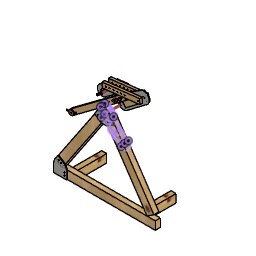
trebuchetAbril2025-Comps-v14 (Autodesk Fusion 360 design; units mm, degrees)
Autodesk Fusion 360 part; units mm, degrees
sketch "Boceto1" plane through (0, 0, 0) normal (0, 1, 0) x (1, 0, 0)
  line L0 (0, 0) -> (800, 0)
  line L1 (800, 0) -> (800, -65)
  line L2 (800, -65) -> (0, -65)
  line L3 (0, -65) -> (0, 0)
  line L4 (65, -65) -> (11.0416, -101.2421)
  line L5 (11.0416, -101.2421) -> (346.0416, -600)
  line L6 (346.0416, -600) -> (400, -563.7579)
  line L7 (400, -563.7579) -> (65, -65)
  line L8 (400, -65) -> (400, -814.7685) construction
  line L9 (400, -563.7579) -> (735, -65)
  line L10 (735, -65) -> (788.9584, -101.2421)
  line L11 (788.9584, -101.2421) -> (453.9584, -600)
  line L12 (453.9584, -600) -> (400, -563.7579)
  dimension "grosor3p" = 65
  dimension "d4" = 65
  dimension "d5" = 600
  dimension "d6" = 65
  dimension "tolerancia" = 1
  dimension "eje" = 10
  dimension "grosorR1b" = 20
  dimension "separacionAgujeros" = 30
  dimension "agujeroAjuste" = 10
  dimension "grosorR2" = 30
  dimension "agujeroTornillos" = 4
  constraint horizontal L0
  constraint vertical L1
  constraint horizontal L2
  constraint vertical L3
  constraint coincident L0.start L3.end
  constraint perpendicular L4 L5
  constraint parallel L4 L6
  constraint parallel L5 L7
  constraint coincident L2 L4.start
  constraint midpoint L2 L8.start
  constraint perpendicular L2 L8
  constraint coincident L6.end L8
  constraint symmetric L4.start L8 L9.end
  constraint symmetric L4.end L8 L10.end
  constraint symmetric L5.end L8 L11.end
  constraint symmetric L6.end L8 L7.start
  measures "grosor3p" distance of L0.start L2.end
  measures "d4" distance of L5 L7
  measures "d5" distance of L0 L5.end
  measures "d6" distance of L2.end L4.start
sketch "Boceto2" plane through (0, 0, 0) normal (0, 1, 0) x (1, 0, 0)
  line L0 (-333.2779, 0) -> (-245.9669, 0)
  line L1 (-245.9669, 0) -> (-245.9669, -600)
  line L2 (-245.9669, -600) -> (-333.2779, -600)
  line L3 (-333.2779, -600) -> (-333.2779, 0)
  constraint horizontal L0
  constraint vertical L1
  constraint horizontal L2
  constraint vertical L3
extrude "Extruir1" add sketch "Boceto1" along normal blind 40 contours L0 L1 L2 L3 | L4 L5 L6 L7 | L9 L10 L11 L12 makes body 1
sketch "Boceto3" plane through (0, 0, 0) normal (0, -1, 0) x (1, 0, 0)
  line L0 (65, 65) -> (400, 563.7579)
  line L1 (400, 563.7579) -> (346.0416, 600)
  line L2 (346.0416, 600) -> (11.0416, 101.2421)
  line L3 (11.0416, 101.2421) -> (65, 65)
  circle A0 centre (65, 65) radius 65
  line L4 (0, 0) -> (105, 0)
  line L5 (105, 0) -> (105, 63.8522)
  line L6 (105, 63.8522) -> (0, 63.8522)
  line L7 (0, 63.8522) -> (0, 0)
  line L8 (65, 65) -> (11.0416, 101.2421)
  line L9 (11.0416, 101.2421) -> (33.3445, 134.4473)
  line L10 (33.3445, 134.4473) -> (87.3029, 98.2052)
  line L11 (87.3029, 98.2052) -> (65, 65)
  circle A1 centre (400, 600) radius 44.7924
  line L12 (0, 0) -> (800, 0)
  line L13 (788.9584, 101.2421) -> (453.9584, 600)
  line L14 (323.7388, 566.7948) -> (377.6971, 530.5527)
  line L15 (377.6971, 530.5527) -> (416.7749, 588.7328)
  line L16 (416.7749, 588.7328) -> (362.8165, 624.975)
  line L17 (362.8165, 624.975) -> (323.7388, 566.7948)
  line L18 (422.7884, 530.8788) -> (476.2612, 566.7948)
  line L19 (476.2612, 566.7948) -> (437.1835, 624.975)
  line L20 (437.1835, 624.975) -> (383.7107, 589.059)
  line L21 (383.7107, 589.059) -> (422.7884, 530.8788)
  line L22 (87.3029, 98.2052) -> (105, 63.8522)
  line L23 (377.6971, 530.5527) -> (422.7884, 530.8788)
  dimension "traslape" = 40
  dimension "d10" = 40
  dimension "d11" = 600
  dimension "d12" = 40
  dimension "d13" = 40
  constraint coincident L0.start L3.end
  constraint coincident L2.end A0
  constraint horizontal L4
  constraint vertical L5
  constraint horizontal L6
  constraint vertical L7
  constraint coincident L4.start L7.end
  constraint perpendicular L8 L9
  constraint parallel L8 L10
  constraint parallel L9 L11
  constraint coincident L2.end L3.start
  constraint perpendicular L2 L8
  constraint vertical L0.end A1.centre
  constraint tangent A1 L13
  constraint perpendicular L14 L15
  constraint parallel L14 L16
  constraint parallel L15 L17
  constraint coincident L0 L14.end
  constraint perpendicular L0 L14
  constraint coincident L2 L14.start
  constraint perpendicular L18 L19
  constraint parallel L18 L20
  constraint parallel L19 L21
  constraint coincident L13 L18.end
  constraint perpendicular L13 L18
  constraint coincident A1 L16.end
  constraint coincident A1 L19.end
  measures "traslape" distance of L8 L10
  measures "d10" distance of L0.start L5
  measures "d11" distance of A1.centre L12
  measures "d12" distance of L13.end L18
  measures "d13" distance of L1 L14
extrude "Extruir2" add sketch "Boceto3" along normal blind 6 separate body contours L0 L3 A0 L8 L10 L11 | L0 L3 A0 L6 L8 L11 L22 | L2 A0 L9 L10 | A0 L5 L6 | A0 L4 L6 L7 L12 | L0 L1 L2 A1 L14 L15 L17 | L0 A1 L15 L21 L23 | A0 L4 L5 L12 | L0 L1 A1 L15 | L0 A1 L15 L21 | A1 L13 L18 L19 L21 | L1 A1 L17 | L1 A1 L15 L16 L20 L21 | A1 L15 L16 L20 L21 | A1 L16 L20 | L15 L16 L20 L21 makes body 2 at (35.0034, 0, 21.2841) makes body 3 at (407.5961, 0, 593.6096)
sketch "Boceto4" plane through (0, 40, 0) normal (0, 1, 0) x (-1, 0, 0)
  line L0 (0, 65) -> (-65, 65)
  line L1 (-65, 65) -> (-735, 65)
  line L2 (-735, 65) -> (-800, 65)
  line L3 (-800, 65) -> (-800, 0)
  line L4 (-800, 0) -> (0, 0)
  line L5 (0, 0) -> (0, 65)
  line L6 (-145, 0) -> (-105, 0)
  line L7 (-105, 0) -> (-105, 65)
  line L8 (-105, 65) -> (-145, 65)
  line L9 (-145, 65) -> (-145, 0)
  line L10 (-400, 65) -> (-400, 691.7695) construction
  line L11 (-655, 65) -> (-655, 0)
  line L12 (-695, 65) -> (-655, 65)
  line L13 (-695, 0) -> (-695, 65)
  line L14 (-655, 0) -> (-695, 0)
  dimension "d16" = 40
  dimension "d17" = 105
  constraint horizontal L6
  constraint vertical L7
  constraint horizontal L8
  constraint vertical L9
  constraint coincident L1 L7.end
  constraint coincident L4 L6.start
  constraint midpoint L1 L10.start
  constraint perpendicular L1 L10
  constraint symmetric L6.start L10 L11.end
  constraint symmetric L6.end L10 L13.start
  constraint symmetric L7.end L10 L12.start
  constraint symmetric L8.end L10 L11.start
  measures "d16" distance of L7.end L8.end
  measures "d17" distance of L5 L7
sketch "Boceto5" plane through (0, 0, 0) normal (0, 0, 1) x (1, 0, 0)
  line L0 (-250, 0) -> (-340.1586, 0)
  line L1 (-340.1586, 0) -> (-340.1586, 310)
  line L2 (-340.1586, 310) -> (-250, 310)
  line L3 (-250, 310) -> (-250, 0)
  dimension "base" = 310
  constraint horizontal L0
  constraint vertical L1
  constraint horizontal L2
  constraint vertical L3
  measures "base" distance of L0.end L1.end
extrude "Extruir3" add sketch "Boceto4" along normal blind 230 separate body contours L1 L4 L6 L7 L8 L9 | L1 L4 L11 L12 L13 L14 makes body 4 at (105, 116.6667, 21.6667) makes body 5 at (655, 116.6667, 43.3333)
sketch "Boceto6" plane through (0, -6, 0) normal (0, -1, 0) x (1, 0, 0)
  line L0 (377.6971, 530.5527) -> (422.7884, 530.8788)
  line L1 (422.7884, 530.8788) -> (476.2612, 566.7948)
  line L2 (476.2612, 566.7948) -> (437.1835, 624.975)
  arc A0 (437.1835, 624.975) -> (362.8165, 624.975) centre (400, 600) ccw
  line L3 (362.8165, 624.975) -> (323.7388, 566.7948)
  line L4 (323.7388, 566.7948) -> (377.6971, 530.5527)
  circle A1 centre (400, 600) radius 5.5
  dimension "d21" = 11
  constraint concentric A0 A1
  measures "d21" diameter of A1
extrude "Extruir4" cut sketch "Boceto6" against normal blind 20 contours A1 bodies 3
sketch "Boceto7" plane through (0, -6, 0) normal (0, -1, 0) x (1, 0, 0)
  circle A0 centre (400, 600) radius 5.5
  line L0 (377.6971, 530.5527) -> (422.7884, 530.8788)
  line L1 (422.7884, 530.8788) -> (476.2612, 566.7948)
  line L2 (476.2612, 566.7948) -> (437.1835, 624.975)
  arc A1 (437.1835, 624.975) -> (362.8165, 624.975) centre (400, 600) ccw
  line L3 (362.8165, 624.975) -> (323.7388, 566.7948)
  line L4 (323.7388, 566.7948) -> (377.6971, 530.5527)
  circle A2 centre (400, 600) radius 5
  dimension "d26" = 10
  constraint concentric A0 A2
  measures "d26" diameter of A2
extrude "Extruir5" add sketch "Boceto7" against normal blind 322 separate body contours A2 makes body 6
ref_plane "PlanoDeObra1" through (400, 0, 563.7579) normal (-1, 0, 0) x (0, -1, 0)
ref_plane "PlanoDeObra2" through (400, 155, 600) normal (0, -1, 0) x (1, 0, 0)
sketch "Boceto8" plane through (0, 155, 0) normal (0, -1, 0) x (-1, 0, 0)
  line L0 (80, -615) -> (-460, -615)
  line L1 (-460, -615) -> (-460, -655)
  line L2 (-460, -655) -> (80, -655)
  line L3 (80, -655) -> (80, -615)
  line L4 (-400, -603.6242) -> (-400, -560.1336)
  line L5 (-400, -605) -> (-384, -605) construction
  circle A0 centre (-400, -600) radius 5 construction
  dimension "r1" = 540
  dimension "grosorR1" = 40
  dimension "d45" = 60
  dimension "d46" = 10
  constraint horizontal L0
  constraint vertical L1
  constraint horizontal L2
  constraint vertical L3
  constraint horizontal L5
  constraint tangent L5 A0
  measures "r1" distance of L1.end L2.end
  measures "grosorR1" distance of L0 L2
  measures "d45" distance of L1 L4
  measures "d46" distance of L0 L5
extrude "Extruir6" add sketch "Boceto8" along normal mid plane 20 separate body makes body 7
sketch "Boceto9" plane through (0, 165, 0) normal (0, 1, 0) x (-1, 0, 0)
  line L0 (80, 615) -> (80, 655)
  line L1 (80, 655) -> (-460, 655)
  line L2 (-460, 655) -> (-460, 615)
  line L3 (-460, 615) -> (80, 615)
  line L4 (-460, 635) -> (80, 635) construction
  circle A0 centre (-430, 635) radius 5
  dimension "d36" = 10
  dimension "d37" = 30
  constraint midpoint L2 L4.start
  constraint midpoint L0 L4.end
  constraint coincident L4 A0.centre
  measures "d36" diameter of A0
  measures "d37" distance of L4.start A0.centre
extrude "Extruir7" cut sketch "Boceto9" against normal blind 50 contours A0 bodies 7
pattern_linear "Patrón R1" count 8 spacing 30 along (-1, 0, 0) of "Extruir7"
sketch "Boceto11" plane through (0, 165, 0) normal (0, 1, 0) x (-1, 0, 0)
  circle A0 centre (-220, 635) radius 5
  circle A1 centre (-250, 635) radius 5
  circle A2 centre (-280, 635) radius 5
  circle A3 centre (-310, 635) radius 5
  circle A4 centre (-340, 635) radius 5
  circle A5 centre (-370, 635) radius 5
  circle A6 centre (-400, 635) radius 5
  circle A7 centre (-430, 635) radius 5
  line L0 (80, 615) -> (80, 655)
  line L1 (80, 655) -> (-460, 655)
  line L2 (-460, 655) -> (-460, 615)
  line L3 (-460, 615) -> (80, 615)
  circle A8 centre (-400, 600) radius 45.5 construction
  line L4 (-355, 655) -> (-445, 655)
  line L5 (-445, 655) -> (-445, 615)
  line L6 (-445, 615) -> (-355, 615) construction
  line L7 (-355, 615) -> (-355, 655)
  line L8 (-400, 615) -> (-400, 586.9631) construction
  circle A9 centre (-400, 600) radius 5 construction
  line L9 (-355, 615) -> (-354.5282, 601.6012)
  arc A10 (-437.3382, 573.9979) -> (-354.5282, 601.6012) centre (-400, 600) ccw
  circle A11 centre (-430, 635) radius 5
  circle A12 centre (-400, 635) radius 5
  circle A13 centre (-370, 635) radius 5
  circle A14 centre (-400, 600) radius 5.5
  line L10 (-445, 615) -> (-419.3317, 615) construction
  line L11 (-419.3317, 615) -> (-419.3317, 585) construction
  line L12 (-419.3317, 585) -> (-445, 585) construction
  line L13 (-445, 585) -> (-445, 615)
  line L14 (-445, 585) -> (-437.3382, 573.9979)
  line L15 (-445, 585) -> (-600, 585)
  line L16 (-600, 585) -> (-600, 615)
  line L17 (-600, 615) -> (-445, 615)
  line L18 (-445, 615) -> (-445, 585)
  line L19 (-445, 655) -> (-443.5915, 615)
  circle A15 centre (-600, 600) radius 44
  circle A16 centre (-600, 600) radius 4
  line L20 (-600.33, 556.0012) -> (-400.3412, 554.5013)
  line L21 (-445, 655) -> (-603.0842, 643.8918)
  dimension "d47" = 90
  dimension "d48" = 11
  dimension "d52" = 30
  dimension "d53" = 30
  dimension "r2" = 200
  dimension "ejeContrapeso" = 8
  dimension "d56" = 40
  dimension "d94" = 40
  constraint horizontal L4
  constraint vertical L5
  constraint horizontal L6
  constraint vertical L7
  constraint midpoint L6 L8.start
  constraint perpendicular L6 L8
  constraint coincident A8.centre L8
  constraint concentric A8 A9
  constraint coincident L3 L6.end
  constraint coincident A8 L9.end
  constraint tangent A8 L9
  constraint coincident A8 A10.start
  constraint coincident A8.centre A9.centre
  constraint concentric A9 A14
  constraint horizontal L10
  constraint vertical L11
  constraint horizontal L12
  constraint vertical L13
  constraint tangent A8 L14
  constraint coincident A10.start L14.end
  constraint horizontal L15
  constraint vertical L16
  constraint horizontal L17
  constraint vertical L18
  constraint coincident L17 L19.end
  constraint parallel L9 L19
  constraint midpoint L16 A15.centre
  constraint concentric A15 A16
  constraint coincident A15 L20.start
  constraint coincident A10 L20.end
  constraint tangent A15 L20
  constraint tangent A8 L20
  constraint coincident A15 L21.end
  constraint tangent A15 L21
  constraint coincident L1.end L4
  measures "d47" distance of L5.end L6.end
  measures "d48" diameter of A14
  measures "d52" distance of L5.end L12.end
  measures "d53" distance of L15.end L16.end
  measures "r2" distance of A8.centre L16
  measures "ejeContrapeso" diameter of A16
  measures "d56" distance of A15 A16
  measures "d94" distance of A8 A14
extrude "Extruir8" add sketch "Boceto11" along normal blind 6 separate body contours L3 L9 A10 L13 L14 L18 | L1 L3 L4 L7 L19 | L3 L5 L19 | L2 L3 L5 L17 L21 | L3 L13 L15 L17 L18 A15 | A10 L14 L15 A15 L20 | L2 L17 A15 L21 | L15 L16 L17 A15 A16 | L15 L16 L17 A15 A16 makes body 8
sketch "Boceto12" plane through (0, 165, 0) normal (0, -1, 0) x (1, 0, 0)
  circle A0 centre (600, 600) radius 4
  circle A1 centre (400, 600) radius 5.5
  arc A2 (600.33, 556.0012) -> (603.0842, 643.8918) centre (600, 600) ccw
  line L0 (445, 655) -> (355, 655)
  line L1 (355, 655) -> (355, 615)
  line L2 (355, 615) -> (354.5282, 601.6012)
  arc A3 (354.5282, 601.6012) -> (400.3412, 554.5013) centre (400, 600) ccw
  line L3 (580, 615) -> (620, 615)
  line L4 (620, 615) -> (620, 315)
  line L5 (620, 315) -> (580, 315)
  line L6 (580, 315) -> (580, 615)
  line L7 (600, 600) -> (600, 505.852) construction
  line L8 (600, 615) -> (600, 315) construction
  line L9 (400.3412, 554.5013) -> (600.33, 556.0012)
  line L10 (603.0842, 643.8918) -> (445, 655)
  circle A4 centre (400, 635) radius 5
  circle A5 centre (430, 635) radius 5
  circle A6 centre (370, 635) radius 5
  dimension "grosorR3" = 40
  dimension "d58" = 15
  dimension "r3a" = 300
  constraint horizontal L3
  constraint vertical L4
  constraint horizontal L5
  constraint vertical L6
  constraint coincident A0.centre A2.centre
  constraint vertical L7
  constraint midpoint L3 L8.start
  constraint midpoint L5 L8.end
  constraint vertical A0.centre L8.start
  measures "grosorR3" distance of L3.start L3.end
  measures "d58" distance of L3 A0.centre
  measures "r3a" distance of L3.end L4.end
extrude "Extruir9" add sketch "Boceto12" along normal blind 20 separate body contours A2 L3 L4 L6 L9 | A2 L4 L5 L6 L9 makes body 9
sketch "Boceto13" plane through (0, 165, 0) normal (0, 1, 0) x (-1, 0, 0)
  line L0 (-620, 615) -> (-620, 315)
  line L1 (-620, 315) -> (-580, 315)
  line L2 (-580, 315) -> (-580, 615)
  circle A0 centre (-600, 345) radius 5
  circle A1 centre (-600, 600) radius 4
  line L3 (-600, 345) -> (-600, 681.8802) construction
  dimension "d62" = 10
  dimension "d63" = 30
  constraint coincident A0.centre L3.start
  constraint coincident A1.centre L3
  measures "d62" diameter of A0
  measures "d63" distance of L1 A0.centre
extrude "Extruir10" cut sketch "Boceto13" against normal blind 35 contours A0 bodies 9 8
pattern_linear "Patrón R2" count 6 spacing 30 along (0, 0, 1) of "Extruir10"
sketch "Boceto14" plane through (0, 165, 0) normal (0, 1, 0) x (-1, 0, 0)
  line L0 (-620, 615) -> (-620, 315)
  line L1 (-620, 315) -> (-580, 315)
  line L2 (-580, 315) -> (-580, 615)
  circle A0 centre (-600, 345) radius 5
  circle A1 centre (-600, 375) radius 5
  circle A2 centre (-600, 405) radius 5
  circle A3 centre (-600, 435) radius 5
  circle A4 centre (-600, 465) radius 5
  circle A5 centre (-600, 495) radius 5
  line L3 (-620, 420) -> (-580, 420)
  line L4 (-580, 420) -> (-580, 330)
  line L5 (-580, 330) -> (-620, 330)
  line L6 (-620, 330) -> (-620, 420)
  line L7 (-600, 420) -> (-600, 330) construction
  line L8 (-620, 375) -> (-580, 375) construction
  line L9 (-648.9711, 369.8205) -> (-580, 330) construction
  line L10 (-580, 330) -> (-665.5144, 181.8847)
  line L11 (-665.5144, 181.8847) -> (-734.4856, 221.7052)
  line L12 (-734.4856, 221.7052) -> (-648.9711, 369.8205)
  line L13 (-648.9711, 369.8205) -> (-620, 420)
  circle A6 centre (-700, 201.7949) radius 12.5
  circle A7 centre (-700, 201.7949) radius 39.8205
  circle A8 centre (-600, 600) radius 4
  line L14 (-580, 615) -> (-620, 615)
  dimension "d71" = 90
  dimension "anguloCodo" = 30
  dimension "d73" = 200
  dimension "ejeMancuerna" = 25
  constraint horizontal L3
  constraint vertical L4
  constraint horizontal L5
  constraint vertical L6
  constraint midpoint L3 L7.start
  constraint midpoint L5 L7.end
  constraint coincident L0 L3.start
  constraint coincident L2 L3.end
  constraint midpoint L6 L8.start
  constraint midpoint L4 L8.end
  constraint coincident A1.centre L8
  constraint perpendicular L9 L10
  constraint parallel L9 L11
  constraint parallel L10 L12
  constraint coincident L4.end L5.start
  constraint perpendicular L9 L13
  constraint coincident L6 L3.start
  constraint coincident L3.start L13
  constraint midpoint L11 A6.centre
  constraint concentric A6 A7
  constraint tangent L12 A7
  measures "d71" distance of L3.end L4.end
  measures "anguloCodo" angle of L5 L9
  measures "d73" distance of A1.centre L11
  measures "ejeMancuerna" diameter of A6
extrude "Extruir11" add sketch "Boceto14" along normal blind 6 separate body contours L0 L2 L3 L4 L5 L6 | L0 L1 L6 L10 L12 L13 A7 | L0 L1 L5 L10 | L11 A6 A7 | L11 A6 A7 makes body 10
sketch "Boceto15" plane through (0, -6, 0) normal (0, -1, 0) x (1, 0, 0)
  arc A0 (11.0416, 101.2421) -> (0.0101, 63.8522) centre (65, 65) ccw
  line L0 (0.0101, 63.8522) -> (0, 63.8522)
  line L1 (0, 63.8522) -> (0, 0)
  line L2 (0, 0) -> (105, 0)
  line L3 (105, 0) -> (105, 63.8522)
  line L4 (105, 63.8522) -> (87.3029, 98.2052)
  line L5 (87.3029, 98.2052) -> (33.3445, 134.4473)
  line L6 (33.3445, 134.4473) -> (11.0416, 101.2421)
  line L7 (11.3477, 125.1292) -> (87.8818, 73.7237)
  line L8 (85, -20) -> (85, 75)
  line L9 (85, 43.3333) -> (140, 43.3333)
  line L10 (85, 21.6667) -> (140, 21.6667)
  line L11 (735, 65) -> (65, 65)
  line L12 (40.1792, 105.764) -> (73.6857, 155.6495)
  line L13 (58.1653, 93.6833) -> (86.3914, 135.7071)
  line L14 (11.0416, 101.2421) -> (346.0416, 600)
  line L15 (400, 563.7579) -> (65, 65)
  line L16 (318.5197, 594.3929) -> (404.0875, 536.9198)
  line L17 (315.6749, 515.9301) -> (352.8763, 571.3167)
  line L18 (342.8096, 517.4701) -> (370.8624, 559.236)
  line L19 (323.7388, 566.7948) -> (377.6971, 530.5527)
  line L20 (400, 603.6242) -> (400, 560.1336)
  line L21 (484.3251, 515.9301) -> (447.1237, 571.3167)
  line L22 (457.1904, 517.4701) -> (429.1376, 559.236)
  line L23 (481.4803, 594.3929) -> (395.9125, 536.9198)
  dimension "d79" = 20
  dimension "d80" = 20
  dimension "d81" = 21.6667
  dimension "d82" = 21.6667
  dimension "d83" = 21.6667
  dimension "d84" = 21.6667
  dimension "d87" = 20
  dimension "d88" = 21.6667
  dimension "d89" = 21.6667
  constraint parallel L5 L7
  constraint parallel L3 L8
  constraint coincident L8 L9.start
  constraint coincident L8 L10.start
  constraint parallel L9 L11
  constraint parallel L10 L11
  constraint coincident L7 L12.start
  constraint coincident L7 L13.start
  constraint parallel L12 L14
  constraint parallel L13 L15
  constraint parallel L14 L17
  constraint parallel L17 L18
  constraint parallel L16 L19
  constraint coincident L16 L17.end
  constraint coincident L16 L18.end
  constraint symmetric L16.start L20 L23.start
  constraint symmetric L16.end L20 L23.end
  constraint symmetric L17.start L20 L21.start
  constraint symmetric L17.end L20 L21.end
  constraint symmetric L18.start L20 L22.start
  constraint symmetric L18.end L20 L22.end
  measures "d79" distance of L5 L7
  measures "d80" distance of L3 L8
  measures "d81" distance of L9 L11
  measures "d82" distance of L9 L10
  measures "d83" distance of L12 L14
  measures "d84" distance of L12 L13
  measures "d87" distance of L16 L19
  measures "d88" distance of L14 L17
  measures "d89" distance of L17 L18
hole "Agujero2" at (40.1792, -6, 105.764) at (58.1653, -6, 93.6833) at (85, -6, 43.3333) at (85, -6, 21.6667) at (352.8763, -6, 571.3167) at (370.8624, -6, 559.236) at (429.1376, -6, 559.236) at (447.1237, -6, 571.3167) direction (0, 1, 0) diameter 10 depth 6 tip angle 180 bodies 2 3
sketch "Boceto16" plane through (0, 165, 0) normal (0, -1, 0) x (1, 0, 0)
  circle A0 centre (430, 635) radius 5
  circle A1 centre (600, 600) radius 4
  circle A2 centre (370, 635) radius 5
  circle A3 centre (400, 635) radius 5
  circle A4 centre (400, 600) radius 5.5
  line L0 (355, 655) -> (355, 615)
  line L1 (355, 615) -> (354.5282, 601.6012)
  arc A5 (354.5282, 601.6012) -> (400.3412, 554.5013) centre (400, 600) ccw
  line L2 (400.3412, 554.5013) -> (600.33, 556.0012)
  arc A6 (600.33, 556.0012) -> (603.0842, 643.8918) centre (600, 600) ccw
  line L3 (603.0842, 643.8918) -> (445, 655)
  line L4 (445, 655) -> (355, 655)
  line L5 (458.2903, 574.9849) -> (578.2903, 575.885)
  line L6 (578.2903, 575.885) -> (577.9903, 615.885)
  line L7 (577.9903, 615.885) -> (457.9903, 614.9849)
  line L8 (457.9903, 614.9849) -> (458.2903, 574.9849)
  line L9 (622.4159, 296.1745) -> (657.0569, 316.1745)
  line L10 (657.0569, 316.1745) -> (717.0569, 212.2514)
  line L11 (717.0569, 212.2514) -> (682.4159, 192.2514)
  line L12 (682.4159, 192.2514) -> (622.4159, 296.1745)
  line L13 (734.4856, 221.7052) -> (620, 420)
  line L14 (580, 330) -> (665.5144, 181.8847)
  line L15 (719.9103, 167.3093) -> (600, 375) construction
  arc A7 (665.5144, 181.8847) -> (734.4856, 221.7052) centre (700, 201.7949) ccw construction
  circle A8 centre (600, 375) radius 5 construction
  line L16 (639.7364, 306.1745) -> (630.415, 322.3197) construction
  point P0 (460, 615)
  dimension "d95" = 40
  dimension "unionMdf" = 120
  dimension "d99" = 40
  dimension "d100" = 120
  constraint perpendicular L5 L6
  constraint parallel L5 L7
  constraint parallel L6 L8
  constraint parallel L2 L5
  constraint coincident L7 P0
  constraint perpendicular L9 L10
  constraint parallel L9 L11
  constraint parallel L10 L12
  constraint parallel L10 L13
  constraint coincident L15.start A7
  constraint coincident L15 A7.centre
  constraint coincident L15.end A8.centre
  constraint midpoint L9 L16.start
  constraint perpendicular L9 L16
  constraint coincident L15 L16.start
  measures "d95" vertical distance of L5.start L7.end
  measures "unionMdf" horizontal distance of L6.end L7.end
  measures "d99" distance of L9.start L9.end
  measures "d100" distance of L9 L11
extrude "Extruir12" add sketch "Boceto16" along normal blind 20 separate body contours L5 L6 L7 L8 | L9 L10 L11 L12 makes body 11 at (538.1903, 165, 588.9183) makes body 12 at (673.9629, 165, 233.5591)
sketch "Boceto17" plane through (0, 171, 0) normal (0, 1, 0) x (-1, 0, 0)
  circle A0 centre (-430, 635) radius 5
  circle A1 centre (-600, 600) radius 4
  circle A2 centre (-370, 635) radius 5
  circle A3 centre (-400, 635) radius 5
  circle A4 centre (-400, 600) radius 5.5
  line L0 (-355, 615) -> (-355, 655)
  line L1 (-355, 655) -> (-445, 655)
  line L2 (-445, 655) -> (-603.0842, 643.8918)
  arc A5 (-603.0842, 643.8918) -> (-600.33, 556.0012) centre (-600, 600) ccw
  line L3 (-600.33, 556.0012) -> (-400.3412, 554.5013)
  arc A6 (-400.3412, 554.5013) -> (-354.5282, 601.6012) centre (-400, 600) ccw
  line L4 (-354.5282, 601.6012) -> (-355, 615)
  line L5 (-457.9903, 614.9849) -> (-458.2903, 574.9849) construction
  line L6 (-458.2903, 574.9849) -> (-578.2903, 575.885) construction
  line L7 (-578.2903, 575.885) -> (-577.9903, 615.885) construction
  line L8 (-577.9903, 615.885) -> (-457.9903, 614.9849) construction
  line L9 (-682.4159, 192.2514) -> (-717.0569, 212.2514) construction
  line L10 (-717.0569, 212.2514) -> (-657.0569, 316.1745) construction
  line L11 (-657.0569, 316.1745) -> (-622.4159, 296.1745) construction
  line L12 (-622.4159, 296.1745) -> (-682.4159, 192.2514) construction
  line L13 (-578.1403, 595.885) -> (-458.1403, 594.9849)
  line L14 (-699.7364, 202.2514) -> (-639.7364, 306.1745)
  line L15 (-659.7364, 271.5334) -> (-642.4159, 261.5334)
  line L16 (-679.7364, 236.8924) -> (-662.4159, 226.8924)
  line L17 (-537.9937, 615.2901) -> (-538.1414, 595.585)
  line L18 (-497.9926, 615.285) -> (-498.1426, 595.285)
  dimension "d102" = 40
  dimension "d103" = 40
  dimension "d104" = 40
  dimension "d105" = 40
  constraint midpoint L7 L13.start
  constraint midpoint L5 L13.end
  constraint midpoint L9 L14.start
  constraint midpoint L11 L14.end
  constraint coincident L12 L15.end
  constraint perpendicular L12 L15
  constraint coincident L12 L16.end
  constraint perpendicular L12 L16
  constraint coincident L13 L17.end
  constraint perpendicular L13 L17
  constraint coincident L8 L18.start
  constraint coincident L13 L18.end
  constraint perpendicular L13 L18
  constraint coincident L14 L16.start
  constraint coincident L14 L15.start
  measures "d102" distance of L11 L15
  measures "d103" distance of L15 L16
  measures "d104" distance of L7 L17
  measures "d105" distance of L17 L18
hole "Agujero3" at (538.1414, 171, 595.585) at (498.1426, 171, 595.285) at (679.7364, 171, 236.8924) at (659.7364, 171, 271.5334) direction (0, -1, 0) diameter 10 depth 50 tip angle 180 bodies 8 10
copy_body "Cuerpo - > Comp.1" bodies 12 removing the originals makes body 13 in component "PaloUnionMdfContrapeso"
copy_body "Cuerpo - > Comp.2" bodies 10 removing the originals makes body 14 in component "MdfCodoContrapeso"
copy_body "Cuerpo - > Comp.3" bodies 9 removing the originals makes body 15 in component "BrazoContrapeso"
copy_body "Cuerpo - > Comp.4" bodies 11 removing the originals makes body 16 in component "PaloUnionMdf"
copy_body "Cuerpo - > Comp.5" bodies 8 removing the originals makes body 17 in component "MdfUnionBrazos"
copy_body "Cuerpo - > Comp.6" bodies 7 removing the originals makes body 18 in component "Brazo1"
sketch "Boceto18" plane through (526.9029, 181, -348.8602) normal (0, -1, 0) x (0.661324, 0, 0.7501)
  circle A0 centre (479.9787, 769.8065) radius 5
  circle A1 centre (517.8896, 757.0487) radius 5
  circle A2 centre (650.9626, 696.4406) radius 5
  circle A3 centre (441.5682, 782.7323) radius 12.5
  circle A4 centre (611.2832, 741.4466) radius 5
  circle A5 centre (631.1229, 718.9436) radius 5
  arc A6 (454.2687, 820.4732) -> (428.8677, 744.9915) centre (441.5682, 782.7323) ccw
  line L0 (428.8677, 744.9915) -> (645.8805, 671.9626)
  line L1 (645.8805, 671.9626) -> (675.8845, 698.4156)
  line L2 (675.8845, 698.4156) -> (616.3653, 765.9246)
  line L3 (616.3653, 765.9246) -> (454.2687, 820.4732)
sketch "Boceto19" plane through (0, 0, 0) normal (0, 1, 0) x (1, 0, 0)
  circle A0 centre (1043.3685, -475.1863) radius 7.5
  circle A1 centre (1043.3685, -475.1863) radius 4.5
  dimension "d153" = 9
  dimension "grosorImpresion" = 3
  constraint concentric A0 A1
  measures "d153" diameter of A1
  measures "grosorImpresion" distance of A0 A1
extrude "Extruir13" add sketch "Boceto19" along normal blind 20 separate body makes body 19
copy_body "Cuerpo - > Comp.7" bodies 19 removing the originals makes body 20 in component "SeparadorEjeContrapeso"
sketch "Boceto20" plane through (0, 0, 0) normal (0, 1, 0) x (1, 0, 0)
  circle A0 centre (-40, -710) radius 4.5
  dimension "d161" = 9
  measures "d161" diameter of A0
extrude "Extruir14" add sketch "Boceto20" along normal blind 37 separate body makes body 21
sketch "Boceto21" plane through (0, 0, 0) normal (0, -1, 0) x (1, 0, 0)
  circle A0 centre (-40, 710) radius 4.5
  circle A1 centre (-40, 710) radius 7.5
  dimension "d164" = 15
  constraint concentric A0 A1
  measures "d164" diameter of A1
extrude "Extruir15" add sketch "Boceto21" along normal blind 5 contours A0 | A1 bodies 21
extrude "Extruir16" add 1 faces at (-43.8923, -5, 708.5917) along direction (0, -1, 0) blind 5 draft 30 on bodies 21 bodies 21
copy_body "Cuerpo - > Comp.8" bodies 21 removing the originals makes body 22 in component "topeAjuste"
sketch "Boceto22" plane through (0, 0, 0) normal (0, 1, 0) x (1, 0, 0)
  circle A0 centre (-303.5213, -478.0896) radius 5.5
  circle A1 centre (-263.5213, -478.0896) radius 5.5
  circle A2 centre (-303.5213, -478.0896) radius 8.5
  circle A3 centre (-263.5213, -478.0896) radius 8.5
  line L0 (-303.5213, -483.5896) -> (-263.5213, -483.5896)
  line L1 (-303.5213, -472.5896) -> (-263.5213, -472.5896)
  dimension "d181" = 11
  dimension "d182" = 11
  dimension "d183" = 3
  dimension "d184" = 3
  dimension "d185" = 40
  constraint concentric A0 A2
  constraint concentric A1 A3
  constraint tangent A0 L1
  constraint tangent A1 L1
  constraint tangent A0 L0
  constraint tangent A1 L0
  constraint coincident A1 L0.end
  constraint coincident A0 L0.start
  constraint coincident A0 L1.start
  constraint coincident A1 L1.end
  constraint horizontal L0
  measures "d181" diameter of A0
  measures "d182" diameter of A1
  measures "d183" distance of A1 A3
  measures "d184" distance of A0 A2
  measures "d185" distance of A0.centre A1.centre
extrude "Extruir17" add sketch "Boceto22" along normal blind 72 separate body contours A0 A2 L0 L1 | A0 A2 L0 L1 | A2 A3 L0 L1 | A1 A3 L0 L1 | A1 A3 L0 L1 makes body 23
copy_body "Cuerpo - > Comp.9" bodies 23 removing the originals makes body 24 in component "separadorMdfContrapeso"
sketch "Boceto23" plane through (0, 0, 0) normal (0, 1, 0) x (1, 0, 0)
  circle A0 centre (-250, -230) radius 5.5
  circle A1 centre (-250, -230) radius 8.5
  dimension "d205" = 11
  dimension "d206" = 3
  constraint concentric A0 A1
  measures "d205" diameter of A0
  measures "d206" distance of A0 A1
extrude "Extruir18" add sketch "Boceto23" along normal blind 91 separate body makes body 25
copy_body "Cuerpo - > Comp.10" bodies 25 removing the originals makes body 26 in component "SeparadorEjecentral"
sketch "Boceto24" plane through (0, 0, 0) normal (0, 1, 0) x (1, 0, 0)
  circle A0 centre (-134.0777, -863.8468) radius 20
  line L0 (-136.5777, -823.8468) -> (-131.5777, -823.8468)
  line L1 (-131.5777, -823.8468) -> (-131.5777, -844.0036)
  line L2 (-131.5777, -844.0036) -> (-136.5777, -844.0036)
  line L3 (-136.5777, -844.0036) -> (-136.5777, -823.8468)
  line L4 (-134.0777, -823.8468) -> (-134.0777, -900) construction
  line L5 (-124.9418, -881.6382) -> (-129.6402, -883.3483)
  line L6 (-129.6402, -883.3483) -> (-122.7462, -902.2895)
  line L7 (-122.7462, -902.2895) -> (-118.0477, -900.5794)
  line L8 (-118.0477, -900.5794) -> (-124.9418, -881.6382)
  line L9 (-120.3969, -901.4345) -> (-142.4198, -840.9272) construction
  circle A1 centre (-134.0777, -863.8468) radius 4.5
  dimension "d217" = 40
  dimension "anguloTope" = 20
  dimension "d219" = 5
  dimension "d220" = 5
  dimension "d221" = 40
  dimension "d222" = 40
  dimension "d223" = 9
  constraint horizontal L0
  constraint vertical L1
  constraint horizontal L2
  constraint vertical L3
  constraint midpoint L0 L4.start
  constraint perpendicular L2 L4
  constraint coincident A0.centre L4
  constraint coincident A0 L1.end
  constraint perpendicular L5 L6
  constraint parallel L5 L7
  constraint parallel L6 L8
  constraint midpoint L7 L9.start
  constraint perpendicular L5 L9
  constraint coincident A0.centre L9
  constraint coincident A0 L5.start
  constraint concentric A0 A1
  measures "d217" diameter of A0
  measures "anguloTope" angle of L4 L9
  measures "d219" distance of L1 L3
  measures "d220" distance of L6 L8
  measures "d221" distance of A0.centre L4.start
  measures "d222" distance of A0.centre L9.start
  measures "d223" diameter of A1
extrude "Extruir19" add sketch "Boceto24" along normal blind 6 separate body makes body 27
sketch "Boceto25" plane through (0, 239.4571, 0) normal (0, -1, 0) x (1, 0, 0)
  circle A0 centre (266.6376, 725.8549) radius 5
  circle A1 centre (291.9849, 709.8077) radius 5
  circle A2 centre (317.3323, 693.7606) radius 5
  circle A3 centre (342.6796, 677.7134) radius 5
  circle A4 centre (368.027, 661.6662) radius 5
  circle A5 centre (393.3743, 645.6191) radius 5
  circle A6 centre (418.7217, 629.5719) radius 5
  circle A7 centre (444.069, 613.5247) radius 5
  line L0 (23.8621, 903.2248) -> (2.4659, 869.4284)
  line L1 (2.4659, 869.4284) -> (458.7183, 580.5793)
  line L2 (458.7183, 580.5793) -> (480.1145, 614.3758)
  line L3 (480.1145, 614.3758) -> (23.8621, 903.2248)
  line L4 (13.164, 886.3266) -> (106.2921, 827.3681) construction
  circle A8 centre (30.0623, 875.6285) radius 4
  circle A9 centre (30.0623, 875.6285) radius 20
  dimension "d226" = 8
  dimension "d227" = 20
  constraint midpoint L0 L4.start
  constraint perpendicular L0 L4
  constraint coincident L4 A8.centre
  constraint concentric A8 A9
  constraint coincident L4.start A9
  measures "d226" diameter of A8
  measures "d227" distance of L0 A8.centre
extrude "Extruir1'" cut sketch "Boceto25" against normal blind 50 contours L0 L3 A9 | L0 L1 A9 | A8 sketch seen with x (0.844912, 0, 0.534906) y (0, 1, 0) z (-0.534906, 0, 0.844912) at (382.9786, -94.4571, -120.9093) bodies 18 in component "Brazo1"
copy_body "Cuerpo - > Comp.11" bodies 27 removing the originals makes body 28 in component "CabezalLanzador"
sketch "Boceto26" plane through (0, -6, 0) normal (0, -1, 0) x (1, 0, 0)
  circle A0 centre (85, 43.3333) radius 5
  circle A1 centre (40.1792, 105.764) radius 5
  circle A2 centre (58.1653, 93.6833) radius 5
  circle A3 centre (85, 21.6667) radius 5
  arc A4 (11.0416, 101.2421) -> (0.0101, 63.8522) centre (65, 65) ccw
  line L0 (0.0101, 63.8522) -> (0, 63.8522)
  line L1 (0, 63.8522) -> (0, 0)
  line L2 (0, 0) -> (105, 0)
  line L3 (105, 0) -> (105, 63.8522)
  line L4 (105, 63.8522) -> (87.3029, 98.2052)
  line L5 (87.3029, 98.2052) -> (33.3445, 134.4473)
  line L6 (33.3445, 134.4473) -> (11.0416, 101.2421)
sketch "Boceto27" plane through (0, -6, 0) normal (0, -1, 0) x (1, 0, 0)
  circle A0 centre (429.1376, 559.236) radius 5
  circle A1 centre (352.8763, 571.3167) radius 5
  circle A2 centre (370.8624, 559.236) radius 5
  circle A3 centre (447.1237, 571.3167) radius 5
  circle A4 centre (400, 600) radius 5.5
  line L0 (377.6971, 530.5527) -> (422.7884, 530.8788)
  line L1 (422.7884, 530.8788) -> (476.2612, 566.7948)
  line L2 (476.2612, 566.7948) -> (437.1835, 624.975)
  arc A5 (437.1835, 624.975) -> (362.8165, 624.975) centre (400, 600) ccw
  line L3 (362.8165, 624.975) -> (323.7388, 566.7948)
  line L4 (323.7388, 566.7948) -> (377.6971, 530.5527)
sketch "Boceto28" plane through (0, -6, 0) normal (0, -1, 0) x (1, 0, 0)
  circle A0 centre (355.7225, 753.0352) radius 5
  circle A1 centre (387.4352, 728.6568) radius 5
  circle A2 centre (482.1553, 655.8429) radius 5
  circle A3 centre (323.5919, 777.7349) radius 12.5
  circle A4 centre (493.6114, 628.1164) radius 5
  circle A5 centre (470.6992, 683.5694) radius 5
  arc A6 (347.8609, 809.3052) -> (299.3229, 746.1645) centre (323.5919, 777.7349) ccw
  line L0 (299.3229, 746.1645) -> (480.8551, 606.6158)
  line L1 (480.8551, 606.6158) -> (517.8238, 621.8906)
  line L2 (517.8238, 621.8906) -> (483.4555, 705.07)
  line L3 (483.4555, 705.07) -> (347.8609, 809.3052)
sketch "Boceto30" plane through (0, 0, 0) normal (0, 1, 0) x (1, 0, 0)
  circle A0 centre (505.4328, -510.6329) radius 5
  circle A1 centre (473.9231, -535.2731) radius 5
  circle A2 centre (556.6199, -475.6207) radius 4
  circle A3 centre (400, -600) radius 5.5
  circle A4 centre (445.2594, -608.7516) radius 5
  circle A5 centre (421.7664, -627.4085) radius 5
  circle A6 centre (398.2734, -646.0654) radius 5
  line L0 (398.9648, -671.0558) -> (374.089, -639.7318)
  line L1 (374.089, -639.7318) -> (365.3868, -629.5327)
  arc A7 (371.9717, -564.1578) -> (365.3868, -629.5327) centre (400, -600) ccw
  line L2 (371.9717, -564.1578) -> (529.5157, -440.9601)
  arc A8 (586.3313, -508.0743) -> (529.5157, -440.9601) centre (556.6199, -475.6207) ccw
  line L3 (586.3313, -508.0743) -> (469.4438, -615.0851)
  line L4 (469.4438, -615.0851) -> (398.9648, -671.0558)
component "PaloUnionMdfContrapeso" placed x (1, 0, 0) y (0, 1, 0) z (0, 0, 1) at (512.0042, 99.8135, 67.2193)
component "MdfCodoContrapeso" placed x (-0.924216, 0, -0.38187) y (0, 1, 0) z (0.38187, 0, -0.924216) at (893.4839, -8.6214, 1231.5458)
component "PaloUnionMdf" placed x (0.7831, 0, -0.621896) y (0, 1, 0) z (0.621896, 0, 0.7831) at (-309.7764, -34.6214, 397.6724)
component "MdfUnionBrazos" placed x (0.7831, 0, -0.621896) y (0, 1, 0) z (0.621896, 0, 0.7831) at (-286.3776, -34.6214, 378.8987)
component "BrazoContrapeso" placed x (-0.924216, 0, -0.38187) y (0, 1, 0) z (0.38187, 0, -0.924216) at (882.0278, -8.6214, 1259.2723)
component "Brazo1" placed x (0.7831, 0, -0.621896) y (0, 1, 0) z (0.621896, 0, 0.7831) at (-286.3776, -34.6214, 378.8987)
component "MdfUnionBrazos" placed x (0.7831, 0, -0.621896) y (0, 1, 0) z (0.621896, 0, 0.7831) at (-286.3776, -60.6214, 378.8987)
component "SeparadorEjeContrapeso" placed x (0.7831, 0, -0.621896) y (0, 1, 0) z (0.621896, 0, 0.7831) at (-555.9582, 110.3786, 752.3695)
component "topeAjuste" placed x (1, 0, 0) y (0, 1, 0) z (0, 0, 1) at (0, 0, 0)
component "topeAjuste" placed x (0.7831, 0, -0.621896) y (0, 1, 0) z (0.621896, 0, 0.7831) at (11.544, 104.3786, 46.5319)
component "topeAjuste" placed x (0.7831, 0, -0.621896) y (0, 1, 0) z (0.621896, 0, 0.7831) at (35.037, 104.3786, 27.875)
component "topeAjuste" placed x (1, 0, 0) y (0, 1, 0) z (0, 0, 1) at (40, 0, 0)
component "topeAjuste" placed x (0.7831, 0, -0.621896) y (0, 1, 0) z (0.621896, 0, 0.7831) at (-11.949, 104.3786, 65.1888)
component "topeAjuste" placed x (1, 0, 0) y (0, 1, 0) z (0, 0, 1) at (40, 0, 0)
component "BrazoContrapeso" placed x (-0.924216, 0, -0.38187) y (0, 1, 0) z (0.38187, 0, -0.924216) at (882.0278, -60.6214, 1259.2723)
component "separadorMdfContrapeso" placed x (-0.792817, 0, 0.60946) y (0, 1, 0) z (-0.60946, 0, -0.792817) at (438.1748, 84.3786, 1292.6784)
component "MdfCodoContrapeso" placed x (-0.924216, 0, -0.38187) y (0, 1, 0) z (0.38187, 0, -0.924216) at (893.4839, -86.6214, 1231.5458)
component "SeparadorEjecentral" placed x (0.950085, 0, 0.31199) y (0, 1, 0) z (-0.31199, 0, 0.950085) at (709.279, 13.3786, 459.4778)
component "SeparadorEjecentral" placed x (0.7831, 0, -0.621896) y (0, 1, 0) z (0.621896, 0, 0.7831) at (452.7388, 136.3786, 264.413)
component "CabezalLanzador" placed x (0.316556, 0, 0.948574) y (0, 1, 0) z (-0.948574, 0, 0.316556) at (923.4061, 104.3786, 767.2076)
equation "d = 800 mm"
equation "h = 600 mm"
equation "d4 = grosor3p"
equation "d5 = h"
equation "d6 = grosor3p"
equation "grosor2p = 40 mm"
equation "d10 = traslape"
equation "d11 = h"
equation "d12 = traslape"
equation "d13 = traslape"
equation "grosorMDF = 6 mm"
equation "d16 = grosor2p"
equation "d17 = grosor3p + traslape"
equation "d19 = base - ( grosor2p * 2 )"
equation "d21 = eje + tolerancia"
equation "tolerancia = 1 mm"
equation "eje = 10 mm"
equation "d26 = eje"
equation "d27 = ( base + 2 * grosorMDF ) * -1"
equation "grosorR1b = 20 mm"
equation "d32 = grosorR1b / 2"
equation "separacionAgujeros = 30 mm"
equation "agujeroAjuste = 10 mm"
equation "d36 = agujeroAjuste"
equation "d37 = separacionAgujeros"
equation "cantidadAgujeros = 8"
equation "d41 = cantidadAgujeros"
equation "d43 = ( cantidadAgujeros - 1 ) * separacionAgujeros"
equation "d45 = separacionAgujeros * 2"
equation "d46 = ( grosorR2 - eje ) / 2"
equation "d47 = separacionAgujeros * 3"
equation "d48 = eje + tolerancia"
equation "d49 = grosorMDF"
equation "grosorR2 = 30 mm"
equation "d52 = grosorR2"
equation "d53 = grosorR2"
equation "d56 = grosorR1"
equation "grosorR3 = grosorR1"
equation "d58 = separacionAgujeros / 2"
equation "grosorR3b = grosorR1b"
equation "d62 = agujeroAjuste"
equation "d63 = separacionAgujeros"
equation "d66 = cantidadAgujerosContra"
equation "d68 = ( cantidadAgujerosContra - 1 ) * separacionAgujeros"
equation "cantidadAgujerosContra = 6"
equation "d71 = 3 * separacionAgujeros"
equation "d76 = grosorMDF"
equation "agujeroTornillos = 4 mm"
equation "d79 = traslape / 2"
equation "d80 = traslape / 2"
equation "d81 = grosor3p / 3"
equation "d82 = grosor3p / 3"
equation "d83 = grosor3p / 3"
equation "d84 = grosor3p / 3"
equation "d87 = traslape / 2"
equation "d88 = grosor3p / 3"
equation "d89 = grosor3p / 3"
equation "d91 = grosorMDF"
equation "d92 = agujeroPernos"
equation "d94 = grosorR1"
equation "d95 = grosorR1"
equation "d97 = grosorR1b"
equation "d99 = grosorR1"
equation "d100 = unionMdf"
equation "d102 = unionMdf / 3"
equation "d103 = unionMdf / 3"
equation "d104 = unionMdf / 3"
equation "d105 = unionMdf / 3"
equation "agujeroPernos = 10 mm"
equation "d153 = ejeContrapeso + tolerancia"
equation "d155 = grosorR3b"
equation "d161 = agujeroAjuste - tolerancia"
equation "d162 = grosorR1b + ( grosorMDF * 2 ) + 5 mm"
equation "d164 = agujeroAjuste + 5 mm"
equation "d181 = agujeroPernos + tolerancia"
equation "d182 = agujeroPernos + tolerancia"
equation "d185 = unionMdf / 3"
equation "d186 = ( 3 * grosorR1b ) + ( 2 * grosorMDF )"
equation "d192 = anguloCodo"
equation "d205 = eje + tolerancia"
equation "d207 = ( ( base - ( ( 2 * grosor2p ) + ( 4 * grosorMDF ) + ( grosorR1b ) ) ) / 2 ) - ( 2 * tolerancia )"
equation "d217 = grosorR1"
equation "d221 = grosorR1"
equation "d222 = d221"
equation "d223 = 8 mm + tolerancia"
equation "d227 = grosorR1 / 2"
named bodies: "PalosA", "MdfUnionA", "MdfSoporteEje", "PaloBase1", "PaloBase2", "Eje", "Brazo1", "MdfUnionBrazos", "MdfCodoContrapeso", "BrazoContrapeso", "PaloUnionMdf", "PaloUnionMdfContrapeso", "SeparadorEjeContrapeso", "topeAjuste", "separadorMdfContrapeso", "SeparadorEjecentral", "CabezalLanzador"
